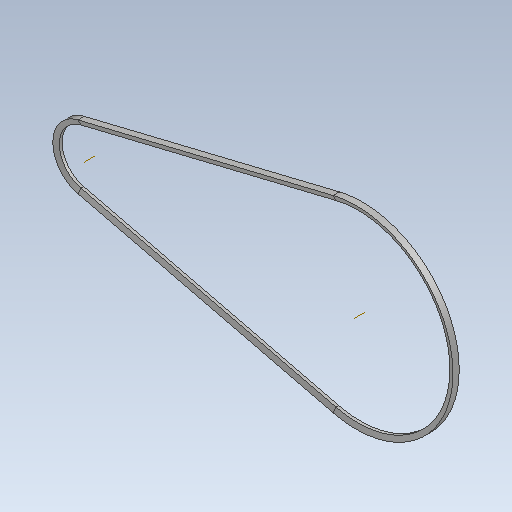
# Autodesk Inventor part: Correa trapezoidal
Saved by Autodesk Inventor 2020 (Build 240168000, 168)
## iProperties
CustomPartVersion: 1
Created: 2021-01-07
Part Number: Correa trapezoidal
Material: Rubber
Document SubType Name: Modeling
Designer: DanielAlvaradoPelaez
Density: 0.93 g/cm^3
Appearance: Rubber - Black - Version 1.1
Author: DanielAlvaradoPelaez
Autodesk Inventor part; units mm, degrees
ref_plane "YZ Plane" through (0, 0, 0) normal (1, 0, 0) x (0, 1, 0)
ref_plane "XZ Plane" through (0, 0, 0) normal (0, 1, 0) x (-1, 0, 0)
ref_plane "XY Plane" through (0, 0, 0) normal (0, 0, 1) x (1, 0, 0)
sketch "Trayectoria de boceto" plane through (0, 0, 0) normal (0, 0, 1) x (1, 0, 0)
  arc A0 (-15.6189, 64.1253) -> (-15.6189, -64.1253) centre (0, 0) ccw
  arc A1 (518.9074, -194.319) -> (518.9074, 194.319) centre (566.2374, 0) ccw
  line L0 (518.9074, -194.319) -> (-15.6189, -64.1253)
  line L1 (-15.6189, 64.1253) -> (518.9074, 194.319)
  constraints: 4 end point, 4 point on circle, 2 centre point
ref_plane "Plano de sección transversal" through (-15.6189, -64.1253, 0) normal (0.971595, -0.2366499, 0) x (0, 0, 1)
sketch "Sección transversal" plane through (-15.6189, -64.1253, 0) normal (0.971595, -0.2366499, 0) x (0, 0, 1)
  line L0 (0, 2.8648) -> (0, -7.1352) construction
  line L1 (-5.5, 0) -> (5.5, 0) construction
  line L2 (-6.5427, 2.8648) -> (6.5427, 2.8648)
  line L3 (6.5427, 2.8648) -> (2.903, -7.1352)
  line L4 (2.903, -7.1352) -> (-2.903, -7.1352)
  line L5 (-2.903, -7.1352) -> (-6.5427, 2.8648)
  point P0 (0, 0)
  point P1 (0, 0)
  point P2 (0, 0)
  dimension "d0" = 11
  dimension "d1" = 2.8648
  dimension "d2" = 40
  dimension "d3" = 10
  constraints: 12 end point, 3 midpoint, 2 parallel, 2 point on line, 1 coincident, 1 perpendicular, 1 vertical, 1 other
  measures "d0" distance of L1.start L1.end
  measures "d1" distance between parallel lines of L2 L1
  measures "d2" angle of L5 L3
  measures "d3" distance between parallel lines of L4 L2
sweep "Correa" add profiles "Sección transversal" path "Trayectoria de boceto" path curves L1 A1 L0 A0
equation "\"d0\" = da_Bw"
equation "\"d1\" = da_Hw"
equation "\"d2\" = da_Alfa"
equation "\"d3\" = da_H"
equation "\"da_Alfa\" = 40deg"
equation "\"da_H\" = 10"
equation "\"da_Bw\" = 11"
equation "\"da_Hw\" = 2.86479"
body "Solid1"
